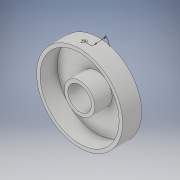
# Autodesk Inventor part: Wheel
Saved by Autodesk Inventor 2017 (Build 210142000, 142)
## iProperties
Created: 2020-02-14
Part Number: Wheel
Material: Generic
Document SubType Name: Modeling
Designer: 10042265
Density: 1 g/cm^3
Appearance: Default
Author: 10042265
Autodesk Inventor part; units mm, degrees
ref_plane "YZ Plane" through (0, 0, 0) normal (1, 0, 0) x (0, 1, 0)
ref_plane "XZ Plane" through (0, 0, 0) normal (0, 1, 0) x (-1, 0, 0)
ref_plane "XY Plane" through (0, 0, 0) normal (0, 0, 1) x (1, 0, 0)
sketch "Sketch1" plane through (0, 0, 0) normal (0, 0, 1) x (1, 0, 0)
  circle A0 centre (0, 0) radius 5.588
  circle A1 centre (0, 0) radius 4.318
  circle A2 centre (0, 0) radius 14.478
  circle A3 centre (0, 0) radius 15.748
  dimension "d1" = 11.176
  dimension "d2" = 1.27
  dimension "d3" = 8.89
  dimension "d4" = 1.27
  constraints: 4 centre point, 1 coincident
  measures "d1" diameter of A0
  measures "d2" radial gap between concentric circles of A0 A1
  measures "d3" radial gap between concentric circles of A0 A2
  measures "d4" radial gap between concentric circles of A2 A3
extrude "Extrusion1" add sketch "Sketch1" along normal mid plane 6.985
sketch "Sketch5" plane through (0, 0, -3.4925) normal (0, 0, -1) x (-1, 0, 0)
  circle A0 centre (0, 0) radius 14.478 projected
  circle A1 centre (0, 0) radius 15.748 projected
  circle A2 centre (0, 0) radius 4.318 projected
  circle A3 centre (0, 0) radius 5.588 projected
extrude "Extrusion3" add sketch "Sketch5" along normal mid plane 1.27 contours A0 | A3
sketch "Sketch6" plane through (0, 0, -4.1275) normal (0, 0, -1) x (-1, 0, 0)
  circle A0 centre (0, 0) radius 14.478 projected
  arc A1 (-3.1559, 14.1299) -> (3.1559, 14.1299) centre (0, 14.478) ccw
  dimension "d17" = 6.35
  constraints: 5 point on circle, 1 centre point
  measures "d17" diameter of A1
body "Solid1"
